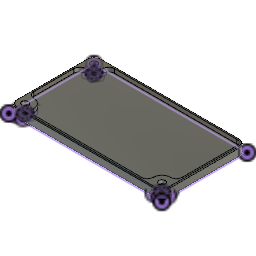
Partie_basse (Autodesk Fusion 360 design; units mm, degrees)
Autodesk Fusion 360 part; units mm, degrees
sketch "Sketch1" plane through (0, 0, 0) normal (0, 0, 1) x (1, 0, 0)
  line L0 (39.5, 22) -> (-39.5, 22)
  line L1 (-39.5, 22) -> (-39.5, -22)
  line L2 (-39.5, -22) -> (39.5, -22)
  line L3 (39.5, -22) -> (39.5, 22)
  line L4 (39.5, 22) -> (-39.5, -22) construction
  line L5 (-39.5, 22) -> (39.5, -22) construction
  dimension "d1" = 44
  dimension "d2" = 79
  constraint horizontal L0
  constraint perpendicular L0 L1
  constraint parallel L0 L2
  constraint parallel L1 L3
  constraint coincident L4 origin
  constraint coincident L5 origin
  measures "d1" distance of L0.end L1.end
  measures "d2" distance of L1.end L2.end
extrude "Extrude1" add sketch "Sketch1" along normal blind 4.5
sketch "Sketch2" plane through (0, 0, 4.5) normal (0, 0, 1) x (-1, 0, 0)
  line L0 (-39.5, 22) -> (-39.5, -22)
  line L1 (-39.5, -22) -> (39.5, -22)
  line L2 (39.5, -22) -> (39.5, 22)
  line L3 (39.5, 22) -> (-39.5, 22)
  line L4 (-38.3, 20.8) -> (-38.3, -20.8)
  line L5 (-38.3, -20.8) -> (38.3, -20.8)
  line L6 (38.3, -20.8) -> (38.3, 20.8)
  line L7 (38.3, 20.8) -> (-38.3, 20.8)
  dimension "d5" = -1.2
extrude "Extrude2" cut sketch "Sketch2" against normal blind 2.1 contours L4 L5 L6 L7
sketch "Sketch3" plane through (0, 0, 2.4) normal (0, 0, 1) x (-1, 0, 0)
  line L0 (38.3, 20.8) -> (-38.3, 20.8)
  line L1 (-38.3, 20.8) -> (-38.3, -20.8)
  line L2 (-38.3, -20.8) -> (38.3, -20.8)
  line L3 (38.3, -20.8) -> (38.3, 20.8)
  line L4 (-38.3, -20.8) -> (-38.3, 20.8)
  line L5 (-38.3, 20.8) -> (38.3, 20.8)
  line L6 (38.3, 20.8) -> (38.3, -20.8)
  line L7 (38.3, -20.8) -> (-38.3, -20.8)
  line L8 (-39.5, 22) -> (-39.5, -22)
  line L9 (-39.5, -22) -> (39.5, -22)
  line L10 (39.5, -22) -> (39.5, 22)
  line L11 (39.5, 22) -> (-39.5, 22)
  circle A0 centre (35.3, -17.8) radius 4.5
  circle A1 centre (-35.3, 17.8) radius 4.5
  circle A2 centre (35.3, 17.8) radius 4.5
  dimension "d8" = 9
  dimension "d9" = 3
  dimension "d10" = 3
  dimension "d11" = 9
  dimension "d12" = 9
  dimension "d13" = 3
  dimension "d14" = 3
  dimension "d15" = 3
  dimension "d16" = 3
  measures "d8" diameter of A0
  measures "d9" distance of L2 A0.centre
  measures "d10" distance of L3 A0.centre
  measures "d11" diameter of A1
  measures "d12" diameter of A2
  measures "d13" distance of L5 A2.centre
  measures "d14" distance of L6 A2.centre
  measures "d15" distance of L1 A1.centre
  measures "d16" distance of L5 A1.centre
extrude "Extrude3" add sketch "Sketch3" along normal blind 2.1 contours L2 L3 L6 L7 A0
extrude "Extrude4" add sketch "Sketch3" along normal blind 2.1 contours L0 L3 L5 L6 A2
extrude "Extrude5" add sketch "Sketch3" along normal blind 2.1 contours L0 L1 L4 L5 A1
sketch "Sketch5" plane through (0, 0, 4.5) normal (0, 0, 1) x (-1, 0, 0)
  line L0 (-38.3, -20.8) -> (-38.3, 14.4459)
  arc A0 (-38.3, 14.4459) -> (-31.9459, 20.8) centre (-35.3, 17.8) ccw
  line L1 (-31.9459, 20.8) -> (31.9459, 20.8)
  arc A1 (31.9459, 20.8) -> (38.3, 14.4459) centre (35.3, 17.8) ccw
  line L2 (38.3, 14.4459) -> (38.3, -14.4459)
  arc A2 (38.3, -14.4459) -> (31.9459, -20.8) centre (35.3, -17.8) ccw
  line L3 (31.9459, -20.8) -> (-38.3, -20.8)
  line L4 (-39.5, 22) -> (-39.5, -22)
  line L5 (-39.5, -22) -> (39.5, -22)
  line L6 (39.5, -22) -> (39.5, 22)
  line L7 (39.5, 22) -> (-39.5, 22)
  circle A3 centre (35.3, -17.8) radius 1.65
  circle A4 centre (35.3, 17.8) radius 1.65
  circle A5 centre (-35.3, 17.8) radius 1.65
  point P0 (35.3, -17.8)
  dimension "d44" = 3.3
  dimension "d45" = 3.3
  dimension "d46" = 3.3
  constraint coincident P0 A2.centre
  constraint concentric A1 A4
  constraint concentric A0 A5
  measures "d44" diameter of A3
  measures "d45" diameter of A4
  measures "d46" diameter of A5
extrude "Extrude7" cut sketch "Sketch5" against normal blind 13 contours A3
extrude "Extrude8" cut sketch "Sketch5" against normal blind 18 contours A4
extrude "Extrude9" cut sketch "Sketch5" against normal blind 16 contours A5
sketch "Sketch6" plane through (0, 0, 0) normal (0, 0, 1) x (1, 0, 0)
  circle A0 centre (35.3, -17.8) radius 1.65
  circle A1 centre (-35.3, -17.8) radius 1.65
  circle A2 centre (-35.3, 17.8) radius 1.65
  line L0 (39.5, 22) -> (39.5, -22)
  line L1 (39.5, -22) -> (-39.5, -22)
  line L2 (-39.5, -22) -> (-39.5, 22)
  line L3 (-39.5, 22) -> (39.5, 22)
  line L4 (-32.1246, -17.8) -> (-33.7123, -15.05)
  line L5 (-33.7123, -15.05) -> (-36.8877, -15.05)
  line L6 (-36.8877, -15.05) -> (-38.4754, -17.8)
  line L7 (-38.4754, -17.8) -> (-36.8877, -20.55)
  line L8 (-36.8877, -20.55) -> (-33.7123, -20.55)
  line L9 (-33.7123, -20.55) -> (-32.1246, -17.8)
  line L10 (-32.1246, 17.8) -> (-33.7123, 20.55)
  line L11 (-33.7123, 20.55) -> (-36.8877, 20.55)
  line L12 (-36.8877, 20.55) -> (-38.4754, 17.8)
  line L13 (-38.4754, 17.8) -> (-36.8877, 15.05)
  line L14 (-36.8877, 15.05) -> (-33.7123, 15.05)
  line L15 (-33.7123, 15.05) -> (-32.1246, 17.8)
  line L16 (32.1246, -17.8) -> (33.7123, -20.55)
  line L17 (33.7123, -20.55) -> (36.8877, -20.55)
  line L18 (36.8877, -20.55) -> (38.4754, -17.8)
  line L19 (38.4754, -17.8) -> (36.8877, -15.05)
  line L20 (36.8877, -15.05) -> (33.7123, -15.05)
  line L21 (33.7123, -15.05) -> (32.1246, -17.8)
  point P0 (-35.3, -17.8)
  point P1 (-35.3, 17.8)
  point P2 (35.3, -17.8)
  dimension "d53" = 2.75
  dimension "d54" = 2.75
  dimension "d55" = 2.75
  constraint coincident P0 A1.centre
  constraint coincident P1 A2.centre
  constraint coincident P2 A0.centre
  constraint horizontal L5
  constraint horizontal L14
  constraint horizontal L20
  measures "d53" distance of P0 L9
  measures "d54" distance of P1 L15
  measures "d55" distance of P2 L21
extrude "Extrude10" cut sketch "Sketch6" along normal blind 2.7 contours L10 L11 L12 L13 L14 L15
extrude "Extrude11" cut sketch "Sketch6" along normal blind 2.7 contours L16 L17 L18 L19 L20 L21
extrude "Extrude12" cut sketch "Sketch6" along normal blind 2.7 contours L4 L5 L6 L7 L8 L9
sketch "Sketch7" plane through (0, 0, 0) normal (0, 0, 1) x (1, 0, 0)
  line L0 (-36.8877, -20.55) -> (-33.7123, -20.55)
  line L1 (-33.7123, -20.55) -> (-32.1246, -17.8)
  line L2 (-32.1246, -17.8) -> (-33.7123, -15.05)
  line L3 (-33.7123, -15.05) -> (-36.8877, -15.05)
  line L4 (-36.8877, -15.05) -> (-38.4754, -17.8)
  line L5 (-38.4754, -17.8) -> (-36.8877, -20.55)
  line L6 (36.8877, -15.05) -> (33.7123, -15.05)
  line L7 (33.7123, -15.05) -> (32.1246, -17.8)
  line L8 (32.1246, -17.8) -> (33.7123, -20.55)
  line L9 (33.7123, -20.55) -> (36.8877, -20.55)
  line L10 (36.8877, -20.55) -> (38.4754, -17.8)
  line L11 (38.4754, -17.8) -> (36.8877, -15.05)
  line L12 (-36.8877, 15.05) -> (-33.7123, 15.05)
  line L13 (-33.7123, 15.05) -> (-32.1246, 17.8)
  line L14 (-32.1246, 17.8) -> (-33.7123, 20.55)
  line L15 (-33.7123, 20.55) -> (-36.8877, 20.55)
  line L16 (-36.8877, 20.55) -> (-38.4754, 17.8)
  line L17 (-38.4754, 17.8) -> (-36.8877, 15.05)
  line L18 (39.5, 22) -> (39.5, -22)
  line L19 (39.5, -22) -> (-39.5, -22)
  line L20 (-39.5, -22) -> (-39.5, 22)
  line L21 (-39.5, 22) -> (39.5, 22)
fillet "Fillet1" radius 3 2 edges at (-31.9459, 20.8, 3.45) (-38.3, 14.4459, 3.45)
fillet "Fillet2" radius 3 2 edges at (-31.9459, -20.8, 3.45) (-38.3, -14.4459, 3.45)
fillet "Fillet3" radius 3 2 edges at (31.9459, -20.8, 3.45) (38.3, -14.4459, 3.45)
fillet "Fillet4" radius 4.2 1 edges at (39.5, -22, 2.25)
fillet "Fillet5" radius 3 1 edges at (38.3, 20.8, 3.45)
fillet "Fillet6" radius 4.2 1 edges at (-39.5, -22, 2.25)
fillet "Fillet7" radius 4.2 1 edges at (-39.5, 22, 2.25)
fillet "Fillet8" radius 4.2 1 edges at (39.5, 22, 2.25)
chamfer "Chamfer1" distance 0.4 angle 45 8 edges at (0, -22, 4.5) (38.2698, -20.7698, 4.5) (39.5, 0, 4.5) (38.2698, 20.7698, 4.5) (0, 22, 4.5) (-38.2698, 20.7698, 4.5) (-39.5, 0, 4.5) (-38.2698, -20.7698, 4.5)
chamfer "Chamfer2" distance 0.4 angle 45 8 edges at (0, -22, 0) (38.2698, -20.7698, 0) (39.5, 0, 0) (38.2698, 20.7698, 0) (0, 22, 0) (-38.2698, 20.7698, 0) (-39.5, 0, 0) (-38.2698, -20.7698, 0)
equation "d53 = ( 5.5 / 2 ) * 1 mm"
equation "d54 = ( 5.5 / 2 ) * 1 mm"
equation "d55 = ( 5.5 / 2 ) * 1 mm"
